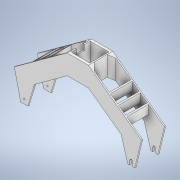
# Autodesk Inventor part: Pont Motor Definitiu
Saved by Autodesk Inventor 2021 (Build 250183000, 183)
## iProperties
Created: 2021-04-15
Part Number: Pont Motor Definitiu
Material: Plástico ABS
Document SubType Name: Modeling
Designer: Marc
Density: 1.06 g/cm^3
Appearance: Suave - Blanco
Author: Marc
## iProperties of the stored document _3DPrint.ipt
Created: 2021-04-16
Part Number: _3DPrint
Material: Genérico
Document SubType Name: Modeling
Designer: Marc
Density: 1 g/cm^3
Appearance: Valor por defecto
Author: Marc
Autodesk Inventor part; units mm, degrees
ref_plane "YZ Plane" through (0, 0, 0) normal (1, 0, 0) x (0, 1, 0)
ref_plane "XZ Plane" through (0, 0, 0) normal (0, 1, 0) x (-1, 0, 0)
ref_plane "XY Plane" through (0, 0, 0) normal (0, 0, 1) x (1, 0, 0)
sketch "Boceto1" plane through (0, 0, 0) normal (0, 0, 1) x (1, 0, 0)
  line L0 (-145, -75) -> (-99, -75)
  line L1 (145, -75) -> (99, -75)
  line L2 (145, -75) -> (145, -13)
  line L3 (-145, -75) -> (-145, -13)
  circle A0 centre (-122, -65) radius 1.6
  circle A1 centre (122, -65) radius 1.6
  line L4 (-24.25, 30) -> (24.25, 30)
  line L5 (0, 75) -> (24.25, 75)
  line L6 (0, 75) -> (-24.25, 75)
  line L7 (-24.25, 75) -> (-145, -13)
  line L8 (24.25, 75) -> (145, -13)
  line L9 (-24.25, 30) -> (-99, -24.4762)
  line L10 (24.25, 30) -> (99, -24.4762)
  line L11 (99, -75) -> (99, -24.4762)
  line L12 (-99, -75) -> (-99, -24.4762)
  dimension "d10" = 3.2
  dimension "d11" = 3.2
  constraints: 26 end point, 4 horizontal, 2 centre point, 1 parallel, 1 vertical
  measures "d10" diameter of A0
  measures "d11" diameter of A1
extrude "Extrusión1" add sketch "Boceto1" along normal blind 55.5
sketch "Boceto7" plane through (0, 0, 55.5) normal (0, 0, 1) x (1, 0, 0)
  circle A0 centre (122, -65) radius 1.6 projected
  arc A1 (125, -65) -> (119, -65) centre (122, -65) ccw
  arc A2 (124.7975, -75) -> (125, -65) centre (-122, -65) ccw
  arc A3 (118.7924, -75) -> (119, -65) centre (-122, -65) ccw
  line L0 (99, -75) -> (145, -75) projected
  line L1 (118.7924, -75) -> (124.7975, -75)
  constraints: 6 point on circle, 3 centre point, 3 coincident, 2 end point, 2 point on line, 1 tangent
extrude "Extrusión7" cut sketch "Boceto7" against normal blind 55.5 contours A0 | A2 L0 A3 A1
sketch "Boceto8" plane through (-24.25, 75, 0) normal (0, 1, 0) x (1, 0, 0)
  line L0 (-120.75, 0) -> (-120.75, -55.5) projected
  line L1 (169.25, 0) -> (169.25, -55.5) projected
  line L2 (24.25, -6) -> (48.5, -6)
  line L3 (48.5, -6) -> (48.5, -3)
  line L4 (48.5, -3) -> (169.25, -3)
  line L5 (24.25, -6) -> (0, -6)
  line L6 (0, -6) -> (0, -3)
  line L7 (0, -3) -> (-120.75, -3)
  line L8 (-120.75, -3) -> (-120.75, -51.5)
  line L9 (169.25, -3) -> (169.25, -52.5)
  line L10 (-120.75, -51.5) -> (-120.75, -52.5)
  line L11 (-120.75, 0) -> (-120.75, -55.5) projected
  line L12 (-120.75, -52.5) -> (0, -52.5)
  line L13 (0, 0) -> (0, -55.5) projected
  line L14 (0, -52.5) -> (0, -49.5)
  line L15 (0, -49.5) -> (48.5, -49.5)
  line L16 (48.5, -49.5) -> (48.5, -52.5)
  line L17 (48.5, 0) -> (48.5, -55.5) projected
  line L18 (48.5, -52.5) -> (169.25, -52.5)
  line L19 (169.25, 0) -> (169.25, -55.5) projected
  dimension "d67" = 3
  dimension "d68" = 3
  dimension "d90" = 1
  dimension "d91" = 3
  constraints: 28 end point, 9 point on line, 5 perpendicular, 2 collinear
  measures "d67" distance of L2.end L3.end
  measures "d68" distance of L5.end L6.end
  measures "d90" distance of L8.end L10.end
  measures "d91" distance of L12.end L14.end
extrude "Extrusión8" cut sketch "Boceto8" against normal blind 150
sketch "Boceto9" plane through (-24.25, 30, 55.5) normal (0, -1, 0) x (1, 0, 0)
  line L0 (-74.75, 0) -> (0, 0) projected
  line L1 (48.5, -55.5) -> (0, -55.5) projected
  line L2 (0, 0) -> (48.5, 0)
  line L3 (48.5, 0) -> (48.5, -55.5)
  line L4 (48.5, -55.5) -> (0, -55.5)
  line L5 (0, -55.5) -> (0, 0)
  circle A0 centre (24.25, -27.25) radius 11.5
  circle A1 centre (8.75, -42.75) radius 2.25
  circle A2 centre (39.75, -42.75) radius 2.25
  circle A3 centre (39.75, -11.75) radius 2.25
  circle A4 centre (8.75, -11.75) radius 2.25
  point P0 (0, -55.5)
  dimension "d71" = 23
  dimension "d75" = 4.5
  dimension "d76" = 4.5
  dimension "d77" = 4.5
  dimension "d78" = 4.5
  constraints: 8 end point, 5 centre point, 2 parallel, 1 horizontal, 1 perpendicular
  measures "d71" diameter of A0
  measures "d75" diameter of A1
  measures "d76" diameter of A2
  measures "d77" diameter of A3
  measures "d78" diameter of A4
extrude "Extrusión9" add sketch "Boceto9" against normal blind 3
sketch "Boceto10" plane through (-24.25, 75, 6) normal (0, 0, 1) x (1, 0, 0)
  line L0 (45.5, 0) -> (45.5, -42)
  line L1 (45.5, -42) -> (48.5, -42)
  line L2 (3, 0) -> (3, -42)
  line L3 (3, -42) -> (0, -42)
  line L4 (3, 0) -> (0, 0)
  line L5 (0, 0) -> (0, -42)
  line L6 (48.5, 0) -> (48.5, -45) projected
  line L7 (45.5, 0) -> (48.5, 0)
  line L8 (48.5, 0) -> (48.5, -42)
  dimension "d81" = 3
  dimension "d82" = 3
  constraints: 16 end point, 1 horizontal, 1 parallel, 1 perpendicular, 1 point on line
  measures "d81" distance of L1.end L0.end
  measures "d82" distance of L2.end L3.end
extrude "Extrusión10" add sketch "Boceto10" along normal blind 43.5
sketch "Boceto13" plane through (-24.25, 75, 3) normal (-1, 0, 0) x (0, 0, 1)
  line L0 (3, 0) -> (46.5, 0) projected
  line L1 (15.75, 0) -> (33.75, 0)
  line L2 (33.75, 0) -> (33.75, -12)
  line L3 (33.75, -12) -> (15.75, -12)
  line L4 (15.75, -12) -> (15.75, 0)
  point P0 (-3, -75)
  dimension "d93" = 18
  dimension "d94" = 12
  constraints: 8 end point, 2 parallel, 1 horizontal, 1 perpendicular, 1 point on line
  measures "d93" distance of L2.end L3.end
  measures "d94" distance of L1.end L2.end
extrude "Extrusión12" cut sketch "Boceto13" against normal blind 3
sketch "Boceto14" plane through (-24.25, 75, 0) normal (0, 1, 0) x (1, 0, 0)
  line L0 (0, -3) -> (-10, -3)
  line L1 (0, -13) -> (0, -3)
  line L2 (48.5, -3) -> (58.5, -3)
  line L3 (48.5, -13) -> (48.5, -3)
  line L4 (-10, -3) -> (0, -13)
  line L5 (0, -42.5) -> (-10, -52.5)
  line L6 (48.5, -13) -> (58.5, -3)
  line L7 (48.5, -42.5) -> (58.5, -52.5)
  line L8 (58.5, -52.5) -> (48.5, -52.5)
  line L9 (48.5, -52.5) -> (48.5, -42.5)
  line L10 (0, -42.5) -> (0, -52.5)
  line L11 (0, -52.5) -> (-10, -52.5)
  constraints: 24 end point, 3 horizontal, 2 perpendicular
extrude "Extrusión13" add sketch "Boceto14" against normal blind 45
sketch "Boceto15" plane through (0, 0, 55.5) normal (0, 0, 1) x (1, 0, 0)
  line L0 (34.25, 75) -> (24.25, 75) projected
  line L1 (24.25, 75) -> (34.25, 75)
  line L2 (34.25, 75) -> (34.25, 67.7122)
  line L3 (34.25, 67.7122) -> (24.25, 75)
  line L4 (-24.25, 75) -> (-34.25, 75) projected
  line L5 (-24.25, 75) -> (-34.25, 75)
  line L6 (-34.25, 75) -> (-34.25, 67.7122) projected
  line L7 (-34.25, 75) -> (-34.25, 67.7122)
  line L8 (-34.25, 67.7122) -> (-24.25, 75)
  point P0 (0, 0)
  constraints: 12 end point, 2 horizontal, 1 collinear, 1 perpendicular
extrude "Extrusión14" cut sketch "Boceto15" against normal blind 55
sketch "Boceto18" plane through (0, 0, 55.5) normal (0, 0, 1) x (1, 0, 0)
  line L0 (-145, -13) -> (-130.4922, -75)
  line L1 (-99, -75) -> (-145, -75) projected
  line L2 (-145, -13) -> (-145, -75) projected
  line L3 (-130.4922, -75) -> (-145, -75)
  line L4 (-145, -75) -> (-145, -13)
  line L5 (-99, -24.4762) -> (-99, -75) projected
  line L6 (-99, -75) -> (-114, -75)
  line L7 (-114, -75) -> (-99, -24.4762)
  line L8 (-99, -24.4762) -> (-99, -75)
  line L9 (99, -24.4762) -> (99, -75) projected
  line L10 (99, -24.4762) -> (99, -75)
  line L11 (99, -75) -> (114, -75)
  line L12 (99, -75) -> (145, -75) projected
  line L13 (24.25, 30) -> (99, -24.4762) projected
  line L14 (114, -75) -> (99, -24.4762)
  line L15 (145, -75) -> (130, -75)
  line L16 (99, -75) -> (145, -75) projected
  line L17 (145, -75) -> (145, -13) projected
  line L18 (130, -75) -> (145, -13)
  line L19 (145, -13) -> (145, -75)
  point P0 (0, 0)
  point P1 (120.1936, -75)
  point P2 (123.3963, -75)
  dimension "d117" = 15
  dimension "d118" = 15
  dimension "d119" = 15
  constraints: 24 end point, 4 point on line, 2 collinear, 2 perpendicular, 1 horizontal
  measures "d117" distance of L1.start L6.end
  measures "d118" distance of L9.end L11.end
  measures "d119" distance of L12.end L15.end
extrude "Extrusión17" cut sketch "Boceto18" against normal blind 55.5
sketch "Boceto19" plane through (122, -65, 52.5) normal (0, 0, -1) x (-1, 0, 0)
  line L0 (97.75, 95) -> (87.75, 95) projected
  line L1 (87.75, 95) -> (87.75, 87.7122)
  line L2 (97.75, 95) -> (23, 40.5238) projected
  line L3 (87.75, 87.7122) -> (97.75, 95)
  line L4 (97.75, 95) -> (87.75, 95)
  line L5 (221, 40.5238) -> (146.25, 95) projected
  line L6 (156.25, 95) -> (146.25, 95) projected
  line L7 (146.25, 95) -> (156.25, 95)
  line L8 (156.25, 95) -> (156.25, 87.7122)
  line L9 (156.25, 87.7122) -> (146.25, 95)
  point P0 (122, 65)
  constraints: 12 end point, 2 perpendicular, 1 collinear, 1 point on line, 1 vertical
extrude "Extrusión18" add sketch "Boceto19" along normal blind 10
sketch "Boceto20" plane through (-34.25, 30, 3) normal (0, 0, 1) x (1, 0, 0)
  line L0 (10, 0) -> (0, 0) projected
  line L1 (0, 0) -> (10, 0)
  line L2 (10, 0) -> (0, -7.2878)
  line L3 (-64.75, -54.4762) -> (10, 0) projected
  line L4 (0, 0) -> (0, -7.2878)
  line L5 (68.5, 0) -> (58.5, 0) projected
  line L6 (133.25, -54.4762) -> (58.5, 0) projected
  line L7 (68.5, 0) -> (58.5, 0)
  line L8 (68.5, 0) -> (68.5, -7.2878)
  line L9 (68.5, 0) -> (58.5, 0) projected
  line L10 (58.5, 0) -> (68.5, -7.2878)
  point P0 (34.25, -30)
  constraints: 12 end point, 2 horizontal, 2 point on line, 1 perpendicular, 1 vertical
extrude "Extrusión19" add sketch "Boceto20" along normal blind 10
sketch "Boceto21" plane through (-34.25, 30, 13) normal (0, 1, 0) x (1, 0, 0)
  line L0 (0, 10) -> (0, 0) projected
  line L1 (10, 0) -> (0, 10) projected
  line L2 (0, 10) -> (10, 0)
  line L3 (10, 0) -> (0, 0) projected
  line L4 (10, 0) -> (0, 0)
  line L5 (0, 0) -> (0, 10)
  line L6 (68.5, 10) -> (58.5, 0) projected
  line L7 (58.5, 0) -> (68.5, 10)
  line L8 (68.5, 10) -> (68.5, 0) projected
  line L9 (68.5, 10) -> (68.5, 0)
  line L10 (58.5, 0) -> (68.5, 0) projected
  line L11 (68.5, 0) -> (58.5, 0)
  line L12 (10, -29.5) -> (0, -39.5)
  line L13 (0, -29.5) -> (10, -29.5) projected
  line L14 (0, -39.5) -> (0, -29.5)
  line L15 (0, -29.5) -> (10, -29.5)
  line L16 (58.5, 0) -> (58.5, -29.5) projected
  line L17 (68.5, -29.5) -> (58.5, -29.5) projected
  line L18 (58.5, -29.5) -> (68.5, -29.5)
  line L19 (68.5, -39.5) -> (68.5, -29.5) projected
  line L20 (68.5, -29.5) -> (68.5, -39.5)
  line L21 (58.5, -29.5) -> (58.5, -42.5) projected
  line L22 (68.5, -39.5) -> (58.5, -29.5)
  line L23 (0, -39.5) -> (0, -29.5) projected
  line L24 (0, -39.5) -> (10, -29.5)
  point P0 (34.25, 13)
  constraints: 26 end point, 7 collinear, 4 perpendicular, 1 point on line
extrude "Extrusión20" cut sketch "Boceto21" against normal blind 10
sketch "Boceto22" plane through (122, -65, 3) normal (0, 0, 1) x (1, 0, 0)
  line L0 (-52.9993, 107.3866) -> (-52.9993, 87.3866)
  line L1 (-52.9993, 87.3866) -> (-50.5748, 85.6197)
  line L2 (-50.5748, 85.6197) -> (-50.5748, 105.6197)
  line L3 (-50.5748, 105.6197) -> (-52.9993, 107.3866)
  line L4 (-34.4116, 93.8404) -> (-34.4116, 73.8404)
  line L5 (-34.4116, 73.8404) -> (-31.9872, 72.0735)
  line L6 (-31.9872, 72.0735) -> (-31.9872, 92.0735)
  line L7 (-31.9872, 92.0735) -> (-34.4116, 93.8404)
  line L8 (-15.824, 80.2941) -> (-15.824, 60.2941)
  line L9 (-15.824, 60.2941) -> (-13.3996, 58.5272)
  line L10 (-13.3996, 58.5272) -> (-13.3996, 78.5272)
  line L11 (-15.824, 80.2941) -> (-13.3996, 78.5272)
  point P0 (-122, 65)
  dimension "d135" = 3
  dimension "d136" = 20
  dimension "d137" = 3
  dimension "d138" = 20
  dimension "d139" = 3
  constraints: 24 end point, 3 parallel, 3 vertical
  measures "d135" distance of L0.end L1.end
  measures "d136" distance of L2.end L4.start
  measures "d137" distance of L4.end L5.end
  measures "d138" distance of L6.end L8.start
  measures "d139" distance of L8.end L9.end
sketch "Boceto23" plane through (-34.25, 22.7122, 3) normal (0, 0, 1) x (1, 0, 0)
  line L0 (10, 52.2878) -> (0, 45) projected
  line L1 (-32.3263, 21.4413) -> (-32.3263, 1.4413)
  line L2 (-32.3263, 1.4413) -> (-34.7507, -0.3256)
  line L3 (-34.7507, -0.3256) -> (-34.7507, 19.6744)
  line L4 (-32.3263, 21.4413) -> (-34.7507, 19.6744)
  line L5 (-50.9139, 7.8951) -> (-50.9139, -12.1049)
  line L6 (-50.9139, -12.1049) -> (-53.3384, -13.8718)
  line L7 (-53.3384, -13.8718) -> (-53.3384, 6.1282)
  line L8 (-50.9139, 7.8951) -> (-53.3384, 6.1282)
  point P0 (34.25, -22.7122)
  dimension "d140" = 40
  dimension "d141" = 20
  dimension "d142" = 3
  dimension "d143" = 20
  dimension "d144" = 3
  constraints: 16 end point, 3 parallel, 2 vertical
  measures "d140" distance of L0.end L1.start
  measures "d141" distance of L1.start L1.end
  measures "d142" distance of L1.end L2.end
  measures "d143" distance of L3.end L5.start
  measures "d144" distance of L5.end L6.end
extrude "Extrusión21" add sketch "Boceto22" along normal blind 49.5
extrude "Extrusión22" add sketch "Boceto23" along normal blind 49.5
sketch "Boceto24" plane through (-34.25, 22.7122, 3) normal (0, 0, 1) x (1, 0, 0)
  line L0 (-69.5015, -5.6512) -> (-69.5015, -25.6512)
  line L1 (-69.5015, -25.6512) -> (-71.926, -27.4181)
  line L2 (-71.926, -27.4181) -> (-71.926, -7.4181)
  line L3 (-71.926, -7.4181) -> (-69.5015, -5.6512)
  point P0 (34.25, -22.7122)
  point P1 (-53.3384, 6.1282)
  dimension "d149" = 20
  dimension "d150" = 20
  dimension "d151" = 3
  constraints: 8 end point, 1 parallel, 1 vertical
  measures "d149" distance of point (-53.338, 6.128) L0.start
  measures "d150" distance of L0.start L0.end
  measures "d151" distance of L0.end L1.end
extrude "Extrusión23" add sketch "Boceto24" along normal blind 49.5
